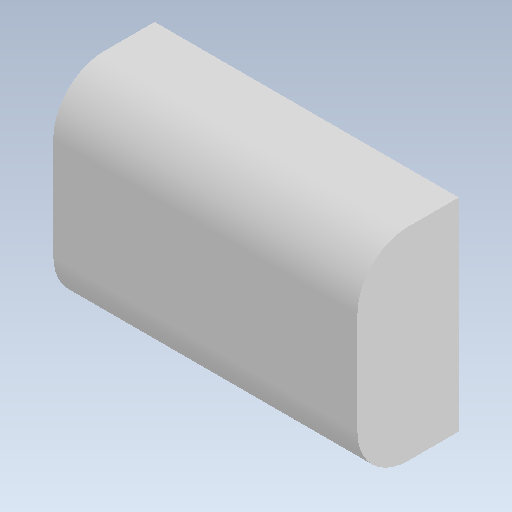
# Autodesk Inventor part: Интвертор
Saved by Autodesk Inventor 2021.2 (Build 252289000, 289)
## iProperties
Created: 2021-10-12
Part Number: Интвертор
Material: Типовые
Document SubType Name: Modeling
Designer: Surflay
Density: 1 g/cm^3
Appearance: По умолчанию
Author: Surflay
Autodesk Inventor part; units mm, degrees
ref_plane "YZ Plane" through (0, 0, 0) normal (1, 0, 0) x (0, 1, 0)
ref_plane "XZ Plane" through (0, 0, 0) normal (0, 1, 0) x (-1, 0, 0)
ref_plane "XY Plane" through (0, 0, 0) normal (0, 0, 1) x (1, 0, 0)
sketch "Эскиз1" plane through (0, 0, 0) normal (0, 0, 1) x (1, 0, 0)
  line L0 (5.2271, -13.5) -> (34.3271, -13.5) projected
  line L1 (15.7271, 7.05) -> (6.6989, 7.05) projected
  line L2 (-4.4915, 7.05) -> (-34.4915, 7.05)
  line L3 (-34.4915, 7.05) -> (-34.4915, -12.95)
  line L4 (-34.4915, -12.95) -> (-4.4915, -12.95)
  line L5 (-4.4915, -12.95) -> (-4.4915, 7.05)
  point P0 (0, 0)
  dimension "d0" = 20
  dimension "d2" = 30
  constraints: 8 end point, 2 parallel, 1 horizontal, 1 perpendicular, 1 point on line
  measures "d0" distance between parallel lines of L2 L4
  measures "d2" distance between parallel lines of L3 L5
extrude "Выдавливание1" add sketch "Эскиз1" along normal blind 10
fillet "Сопряжение1" radius 5 2 edges at (-19.4915, -12.95, 10) (-19.4915, 7.05, 10)
